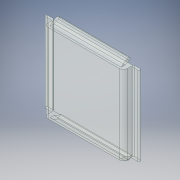
# Autodesk Inventor part: Sight Glass
Saved by Autodesk Inventor 2019 (Build 230136000, 136)
## iProperties
Created: 2019-03-02
Part Number: Sight Glass
Material: Glass
Document SubType Name: Modeling
Designer: User
Density: 2.18 g/cm^3
Appearance: Clear
Author: User
Autodesk Inventor part; units mm, degrees
ref_plane "YZ Plane" through (0, 0, 0) normal (1, 0, 0) x (0, 1, 0)
ref_plane "XZ Plane" through (0, 0, 0) normal (0, 1, 0) x (-1, 0, 0)
sketch "Sketch1" plane through (0, 0, 0) normal (0, 0, 1) x (1, 0, 0)
  line L0 (-50, 50) -> (50, 50)
  line L1 (50, 50) -> (50, -50)
  line L2 (50, -50) -> (-50, -50)
  line L3 (-50, -50) -> (-50, 50)
  line L4 (-50, 50) -> (50, -50) construction
  line L5 (50, 50) -> (-50, -50) construction
  point P0 (0, 0)
  dimension "d0" = 100
  dimension "d1" = 100
  constraints: 12 end point, 2 midpoint, 2 parallel, 1 horizontal, 1 perpendicular
  measures "d0" distance of L1.end L2.end
  measures "d1" distance of L0.end L1.end
extrude "Extrusion1" add sketch "Sketch1" against normal blind 12
sketch "Sketch2" plane through (-50, 50, 0) normal (0, 1, 0) x (1, 0, 0)
  line L0 (0, 0) -> (100, 0) projected
  line L1 (100, 0) -> (100, 12) projected
  line L2 (0, 12) -> (100, 12) projected
  line L3 (0, 0) -> (0, 12) projected
  line L4 (5, 7.5) -> (95, 7.5)
  line L5 (95, 7.5) -> (95, 2.5)
  line L6 (95, 2.5) -> (5, 2.5)
  line L7 (5, 2.5) -> (5, 7.5)
  line L8 (5, 7.5) -> (95, 2.5) construction
  line L9 (95, 7.5) -> (5, 2.5) construction
  point P0 (50, 0)
  point P1 (50, 5)
  dimension "d4" = 90
  dimension "d5" = 5
  constraints: 12 end point, 2 midpoint, 2 parallel, 1 horizontal, 1 perpendicular
  measures "d4" distance of L5.end L6.end
  measures "d5" distance of L4.end L5.end
sketch "Sketch3" plane through (0, 0, 0) normal (1, 0, 0) x (0, 1, 0)
  line L0 (50, 0) -> (50, -12) projected
  arc A0 (53.9199, -14.9331) -> (50, -6) centre (40.9253, -15.3086) ccw
  point P0 (0, 0)
  constraints: 2 point on circle, 1 centre point
sweep "Sweep1" add profiles "Sketch2" path "Sketch3" path curves A0 contours L4 L5 L6 L7
mirror "Mirror1" about plane through (0, 0, 0) normal (0, 1, 0) of "Sweep1"
fillet "Fillet2" radius 5 2 edges at (-50, 0, 0) (50, 0, 0)
ref_plane "Work Plane1" through (0, 0, -10) normal (0, 0, 1) x (1, 0, 0)
sketch "Sketch5" plane through (0, 0, -10) normal (0, 0, 1) x (1, 0, 0)
  line L0 (-50, 50) -> (50, 50) projected
  line L1 (50, 50) -> (60, 50)
  line L2 (60, 50) -> (60, -50)
  line L3 (60, -50) -> (50, -50)
  line L4 (50, -50) -> (50, 50)
  line L5 (-45, 50) -> (45, 50) projected
  line L6 (-50, 50) -> (-60, 50)
  line L7 (-60, 50) -> (-60, -50)
  line L8 (-60, -50) -> (-50, -50)
  line L9 (-50, -50) -> (-50, 50)
  point P0 (0, 0)
  dimension "d17" = 10
  dimension "d18" = 100
  constraints: 16 end point, 2 parallel, 1 horizontal, 1 perpendicular
  measures "d17" distance of L2.end L3.end
  measures "d18" distance of L1.end L2.end
extrude "Extrusion3" add sketch "Sketch5" against normal blind 3
fillet "Fillet3" radius 1.5 6 edges at (-50, 0, -13) (-60, 0, -13) (-60, 0, -10) (60, 0, -13) (50, 0, -13) (60, 0, -10)
fillet "Fillet4" radius 1.5 2 edges at (0, 52.8765, -16.0107) (0, 56.3544, -12.4185)
body "Solid1"
